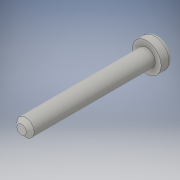
# Autodesk Inventor part: screwKa22x16
Saved by Autodesk Inventor 2016 (Build 200138000, 138)
## iProperties
Created: 2016-06-05
Part Number: screwKa22x16
Material: Generic
Document SubType Name: Modeling
Designer: hesaon
Density: 1 g/cm^3
Appearance: Default
Author: hesaon
Autodesk Inventor part; units mm, degrees
ref_plane "YZ Plane" through (0, 0, 0) normal (1, 0, 0) x (0, 1, 0)
ref_plane "XZ Plane" through (0, 0, 0) normal (0, 1, 0) x (-1, 0, 0)
ref_plane "XY Plane" through (0, 0, 0) normal (0, 0, 1) x (1, 0, 0)
sketch "Sketch1" plane through (0, 0, 0) normal (0, 1, 0) x (-1, 0, 0)
  circle A0 centre (0, 0) radius 1.1
  dimension "d0" = 2.2
  constraints: 1 centre point, 1 coincident
  measures "d0" diameter of A0
extrude "Extrusion1" add sketch "Sketch1" along normal blind 16
sketch "Sketch2" plane through (0, 16, 0) normal (0, 1, 0) x (1, 0, 0)
  circle A0 centre (0, 0) radius 1.85
  dimension "d3" = 3.7
  constraints: 1 centre point, 1 coincident
  measures "d3" diameter of A0
extrude "Extrusion2" add sketch "Sketch2" along normal blind 1.5
fillet "Fillet1" radius 0.5 1 edges at (-1.85, 17.5, 0)
sketch "Sketch3" plane through (0, 17.5, 0) normal (0, 1, 0) x (1, 0, 0)
  line L0 (0.3, -0.9) -> (-0.3, -0.9)
  line L1 (-0.3, 0.9) -> (0.3, 0.9)
  line L2 (0.3, -0.9) -> (-0.3, 0.9) construction
  line L3 (-0.3, -0.9) -> (0.3, 0.9) construction
  line L4 (-0.9, 0.3) -> (-0.9, -0.3)
  line L5 (0.9, -0.3) -> (0.9, 0.3)
  line L6 (0.9, 0.3) -> (-0.9, -0.3) construction
  line L7 (-0.9, 0.3) -> (0.9, -0.3) construction
  line L8 (-0.3, -0.9) -> (-0.3, -0.3)
  line L9 (-0.3, 0.3) -> (-0.3, 0.9)
  line L10 (0.3, 0.9) -> (0.3, 0.3)
  line L11 (0.3, -0.3) -> (0.3, -0.9)
  line L12 (-0.9, -0.3) -> (-0.3, -0.3)
  line L13 (0.3, -0.3) -> (0.9, -0.3)
  line L14 (-0.3, 0.3) -> (-0.9, 0.3)
  line L15 (0.9, 0.3) -> (0.3, 0.3)
  point P0 (0, 0)
  dimension "d7" = 0.6
  dimension "d8" = 1.8
  dimension "d9" = 1.8
  dimension "d10" = 0.6
  dimension "d11" = 0.6
  dimension "d12" = 0.6
  dimension "d13" = 0.6
  dimension "d14" = 0.6
  constraints: 32 end point, 10 parallel, 4 midpoint, 4 perpendicular, 3 horizontal
  measures "d7" distance of L1.start L1.end
  measures "d8" distance of L0.end L1.start
  measures "d9" distance of L5.start L4.end
  measures "d10" distance of L4.end L4.start
  measures "d11" distance of L11.start L8.end
  measures "d12" distance of L10.end L9.start
  measures "d13" distance of L8.end L9.start
  measures "d14" distance of L10.end L11.start
extrude "Extrusion3" cut sketch "Sketch3" against normal blind 1.5
chamfer "Chamfer1" distance 0.5 angle 45 1 edges at (1.1, 0, 0)
body "Solid1"
